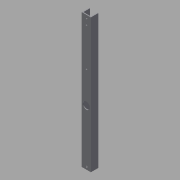
# Autodesk Inventor part: 18in C-Channel Rear
Saved by Autodesk Inventor 2013 (Build 170138000, 138)
## iProperties
Created: 2013-01-08
Part Number: 18in C-Channel Rear
Material: Aluminum 6061
Document SubType Name: Modeling
Designer: Naphat
Density: 1 g/cm^3
Author: Naphat
Autodesk Inventor part; units mm, degrees
ref_plane "YZ Plane" through (0, 0, 0) normal (1, 0, 0) x (0, 1, 0)
ref_plane "XZ Plane" through (0, 0, 0) normal (0, 1, 0) x (-1, 0, 0)
ref_plane "XY Plane" through (0, 0, 0) normal (0, 0, 1) x (1, 0, 0)
sketch "Sketch1" plane through (0, 0, 0) normal (0, 0, 1) x (1, 0, 0)
  line L0 (-15.7, 12.7) -> (-12.7, 12.7)
  line L1 (-12.7, 12.7) -> (-12.7, -9.7)
  line L2 (-12.7, -9.7) -> (12.7, -9.7)
  line L3 (12.7, -9.7) -> (12.7, 12.7)
  line L4 (12.7, 12.7) -> (15.7, 12.7)
  line L5 (15.7, 12.7) -> (15.7, -12.7)
  line L6 (15.7, -12.7) -> (-15.7, -12.7)
  line L7 (-15.7, -12.7) -> (-15.7, 12.7)
  point P0 (0, 0)
  dimension "d0" = 3
  dimension "d2" = 3
  dimension "d3" = 25.4
  dimension "d4" = 31.4
  dimension "d5" = 15.7
  dimension "d7" = 12.7
  dimension "d8" = 3
  constraints: 16 end point, 5 parallel, 1 collinear, 1 horizontal, 1 perpendicular
  measures "d0" distance of L0.start L0.end
  measures "d2" distance of L3.end L4.end
  measures "d3" distance of L6.end L0.start
  measures "d4" distance of L5.end L6.end
  measures "d5" distance from line of point (0, 0) L7
  measures "d7" distance from line of L6 point (0, 0)
  measures "d8" distance between parallel lines of L6 L2
extrude "Extrusion1" add sketch "Sketch1" against normal blind 457.2
sketch "Sketch6" plane through (-15.7, -12.7, 0) normal (0, -1, 0) x (1, 0, 0)
  circle A0 centre (16.6513, -447.9) radius 3.175
  point P0 (15.7, 0)
  dimension "d21" = 6.35
  constraints: 1 centre point
  measures "d21" diameter of A0
extrude "Extrusion4" cut sketch "Sketch6" against normal blind 10
sketch "Sketch7" plane through (-15.7, -12.7, 0) normal (0, -1, 0) x (1, 0, 0)
  line L0 (31.4, -134) -> (0, -134) construction
  line L1 (31.4, -184) -> (0, -184) construction
  line L2 (0, -184) -> (0, -134) construction
  line L3 (0, -159) -> (15.7, -159) construction
  line L4 (15.7, -159) -> (15.7, -184) construction
  circle A0 centre (15.7, -159) radius 3.175
  point P0 (15.7, 0)
  dimension "d25" = 6.35
  constraints: 10 end point, 2 midpoint, 1 centre point, 1 coincident, 1 perpendicular
  measures "d25" diameter of A0
extrude "Extrusion5" cut sketch "Sketch7" against normal blind 10
sketch "Sketch8" plane through (-15.7, -12.7, 0) normal (0, -1, 0) x (1, 0, 0)
  circle A0 centre (16.6513, -9.3) radius 3.175
  circle A1 centre (15.7, -29) radius 3.175
  circle A2 centre (16.6513, -9.3) radius 3.175
  circle A3 centre (15.7, -29) radius 3.175
  circle A4 centre (15.7, -159) radius 3.175
  circle A5 centre (16.6513, -447.9) radius 3.175
  line L0 (31.4, 0) -> (0, 0)
  line L1 (0, 0) -> (0, -457.2)
  line L2 (31.4, -457.2) -> (0, -457.2)
  line L3 (31.4, 0) -> (31.4, -457.2)
  circle A6 centre (15.7, -268.2855) radius 12.1666
  point P0 (15.7, 0)
  point P1 (15.7, 0)
  dimension "d33" = 188.9145
  dimension "d34" = 15.7
  dimension "d35" = 31.4
  constraints: 8 end point, 7 centre point
  measures "d33" distance from line of L2 A6.centre
  measures "d34" distance from line of L1 A6.centre
  measures "d35" distance of L2.start L1.end
extrude "Extrusion6" cut sketch "Sketch8" against normal blind 10 contours A0 | A1 | A6
equation "\"d2\" = d0"
equation "\"d5\" = 0.5 * d4"
equation "\"d7\" = 0.5 * d3"
equation "\"d8\" = d0"
equation "\"d34\" = 0.5 * d35"
body "Solid1"
